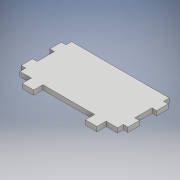
# Autodesk Inventor part: FUENTE 2
Saved by Autodesk Inventor 2018 (Build 220112000, 112)
## iProperties
Created: 2018-03-06
Part Number: FUENTE 2
Material: Generic
Document SubType Name: Modeling
Designer: isai
Density: 1 g/cm^3
Appearance: Default
Author: isai
Autodesk Inventor part; units mm, degrees
ref_plane "YZ Plane" through (0, 0, 0) normal (1, 0, 0) x (0, 1, 0)
ref_plane "XZ Plane" through (0, 0, 0) normal (0, 1, 0) x (-1, 0, 0)
ref_plane "XY Plane" through (0, 0, 0) normal (0, 0, 1) x (1, 0, 0)
sketch "Sketch1" plane through (0, 0, 0) normal (0, 0, 1) x (1, 0, 0)
  line L0 (42.5, -22.5) -> (-42.5, -22.5)
  line L1 (-42.5, -22.5) -> (-42.5, 22.5)
  line L2 (-42.5, 22.5) -> (42.5, 22.5)
  line L3 (42.5, 22.5) -> (42.5, -22.5)
  line L4 (42.5, -22.5) -> (-42.5, 22.5) construction
  line L5 (-42.5, -22.5) -> (42.5, 22.5) construction
  point P0 (0, 0)
  dimension "d0" = 85
  dimension "d1" = 45
  constraints: 12 end point, 2 midpoint, 2 parallel, 1 horizontal, 1 perpendicular
  measures "d0" distance of L1.end L2.end
  measures "d1" distance of L0.end L1.end
extrude "Extrusion1" add sketch "Sketch1" along normal blind 4
sketch "Sketch2" plane through (0, 0, 4) normal (0, 0, 1) x (1, 0, 0)
  line L0 (-42.5, -22.5) -> (42.5, -22.5) projected
  line L1 (42.5, -22.5) -> (42.5, 22.5) projected
  line L2 (42.5, 22.5) -> (-42.5, 22.5) projected
  line L3 (-42.5, 22.5) -> (-42.5, -22.5) projected
  line L4 (42.5, -22.5) -> (42.5, 22.5) projected
  line L5 (42.5, 17.5) -> (46.5, 17.5)
  line L6 (46.5, 17.5) -> (46.5, 7.5)
  line L7 (46.5, 7.5) -> (42.5, 7.5)
  line L8 (42.5, 7.5) -> (42.5, 17.5)
  line L9 (42.5, -7.5) -> (46.5, -7.5)
  line L10 (46.5, -7.5) -> (46.5, -17.5)
  line L11 (46.5, -17.5) -> (42.5, -17.5)
  line L12 (42.5, -17.5) -> (42.5, -7.5)
  point P0 (0, 0)
  dimension "d4" = 4
  dimension "d5" = 10
  dimension "d6" = 4
  dimension "d7" = 10
  dimension "d8" = 5
  dimension "d9" = 5
  constraints: 16 end point, 4 parallel, 2 horizontal, 2 perpendicular, 2 point on line
  measures "d4" distance of L6.end L7.end
  measures "d5" distance of L5.end L6.end
  measures "d6" distance of L10.end L11.end
  measures "d7" distance of L9.end L10.end
  measures "d8" distance between parallel lines of L5 L2
  measures "d9" distance between parallel lines of L11 L0
extrude "Extrusion2" add sketch "Sketch2" against normal blind 4 contours L1 L9 L10 L11 | L5 L6 L7 L1
ref_plane "Work Plane1" through (0, -7.5, 0) normal (1, 0, 0) x (0, 0, -1)
mirror "Mirror1" about plane through (0, -7.5, 0) normal (1, 0, 0) of "Extrusion2"
sketch "Sketch3" plane through (0, 0, 4) normal (0, 0, 1) x (1, 0, 0)
  line L0 (-42.5, -22.5) -> (42.5, -22.5) projected
  line L1 (-32.5, -22.5) -> (-22.5, -22.5)
  line L2 (-22.5, -22.5) -> (-22.5, -30.5)
  line L3 (-22.5, -30.5) -> (-32.5, -30.5)
  line L4 (-32.5, -30.5) -> (-32.5, -22.5)
  line L5 (22.5, -22.5) -> (32.5, -22.5)
  line L6 (32.5, -22.5) -> (32.5, -30.5)
  line L7 (32.5, -30.5) -> (22.5, -30.5)
  line L8 (22.5, -30.5) -> (22.5, -22.5)
  line L9 (-42.5, -17.5) -> (-42.5, -22.5) projected
  line L10 (42.5, -22.5) -> (42.5, -17.5) projected
  point P0 (0, 0)
  dimension "d12" = 10
  dimension "d13" = 8
  dimension "d14" = 10
  dimension "d15" = 8
  constraints: 16 end point, 4 parallel, 2 horizontal, 2 perpendicular, 2 point on line
  measures "d12" distance of L2.end L3.end
  measures "d13" distance of L1.end L2.end
  measures "d14" distance of L6.end L7.end
  measures "d15" distance of L5.end L6.end
extrude "Extrusion3" add sketch "Sketch3" against normal blind 4
equation "\"d5\" = d"
equation "\"d7\" = d"
equation "\"d12\" = d"
equation "\"d14\" = d"
equation "\"d\" = 10"
body "Solid1"
